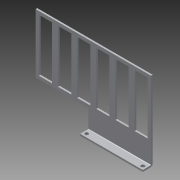
# Autodesk Inventor part: Wall
Saved by Autodesk Inventor 2013 (Build 170138000, 138)
## iProperties
Created: 2013-02-01
Part Number: Wall
Material: Aluminum 6061
Document SubType Name: Sheet Metal
Designer: actoennies
Mass: 272.717 g
Surface Area: 659.98 cm^2
Volume: 100.633 cm^3
Density: 2.71 g/cm^3
Sheet Metal Rule: Default
Author: actoennies
Autodesk Inventor part; units mm, degrees
ref_plane "YZ Plane" through (0, 0, 0) normal (1, 0, 0) x (0, 1, 0)
ref_plane "XZ Plane" through (0, 0, 0) normal (0, 1, 0) x (-1, 0, 0)
ref_plane "XY Plane" through (0, 0, 0) normal (0, 0, 1) x (1, 0, 0)
sketch "Sketch1" plane through (0, 0, 0) normal (0, 1, 0) x (-1, 0, 0)
  line L0 (0, 0) -> (0, 19.05)
  line L1 (0, 19.05) -> (120.65, 19.05)
  line L2 (120.65, 19.05) -> (120.65, 0)
  line L3 (120.65, 0) -> (0, 0)
  circle A0 centre (6.35, 12.7) radius 3.3782
  circle A1 centre (114.3, 12.7) radius 3.3782
  dimension "d0" = 19.05
  dimension "d1" = 120.65
  dimension "d2" = 6.7564
  dimension "d3" = 6.7564
  dimension "d4" = 107.95
  dimension "d5" = 6.35
  dimension "d6" = 12.7
  dimension "d7" = 12.7
  measures "d0" distance of L0.start L0.end
  measures "d1" distance of L0.end L1.end
  measures "d2" diameter of A0
  measures "d3" diameter of A1
  measures "d4" distance of A1.centre A0.centre
  measures "d5" distance from line of L0 A0.centre
  measures "d6" distance from line of L3 A0.centre
  measures "d7" distance from line of L3 A1.centre
extrude "Plate1" add sketch "Sketch1" along normal blind 3.175
sketch "Sketch2" plane through (-120.65, 0, 3.175) normal (0, 0, -1) x (-1, 0, 0)
  line L0 (-120.65, 0) -> (0, 0)
  line L1 (0, 0) -> (0, 38.1)
  line L2 (0, 38.1) -> (-120.65, 38.1)
  line L3 (-120.65, 38.1) -> (-120.65, 0)
  constraints: 6 end point, 1 horizontal, 1 perpendicular, 1 vertical
edge flange "Flange1" height 38.1 angle 90 thickness 3.175 bend radius 1.27 thickness toward (0, 0, -1) relief straight relief width 3.175 relief depth 1.5875 edges at (-60.325, 3.175, 0) wall of the first edge with corners at (0, 0, 3.175) (-120.65, 0, 3.175) (-120.65, 38.1, 3.175) (0, 38.1, 3.175)
bend "Bend1"
corner "Corner1"
sketch "Sketch3" plane through (-120.65, 38.1, 3.175) normal (0, 0, 1) x (1, 0, 0)
  line L0 (120.65, 0) -> (0, 0)
  line L1 (0, 0) -> (0, -33.655)
  line L2 (0, 0) -> (-101.6, 0)
  line L3 (-101.6, 0) -> (-101.6, 114.3)
  line L4 (-101.6, 114.3) -> (120.65, 114.3)
  line L5 (120.65, 114.3) -> (120.65, 0)
  point P0 (120.65, -38.1)
  dimension "d19" = 101.6
  dimension "d20" = 114.3
  measures "d19" distance of L0.end L2.end
  measures "d20" distance of L2.end L3.end
sheet face with bend "Face2" sketch "Sketch3" thickness 3.175 toward (0, 0, -1) bend radius 3.175 relief straight relief width 3.175 relief depth 1.5875
bend "Bend2"
sketch "Sketch4" plane through (-120.65, 4.445, 3.175) normal (0, 0, 1) x (1, 0, 0)
  line L0 (120.65, 147.955) -> (-101.6, 147.955) projected
  line L1 (-101.6, 147.955) -> (-101.6, 33.655) projected
  line L2 (-101.6, 33.655) -> (0, 33.655) projected
  line L3 (0, 33.655) -> (0, 0) projected
  line L4 (-95.25, 141.605) -> (-69.85, 141.605)
  line L5 (-69.85, 141.605) -> (-69.85, 40.005)
  line L6 (-69.85, 40.005) -> (-95.25, 40.005)
  line L7 (-95.25, 40.005) -> (-95.25, 141.605)
  line L8 (-58.42, 141.605) -> (-33.02, 141.605)
  line L9 (-33.02, 141.605) -> (-33.02, 40.005)
  line L10 (-33.02, 40.005) -> (-58.42, 40.005)
  line L11 (-58.42, 40.005) -> (-58.42, 141.605)
  line L12 (-21.59, 141.605) -> (3.81, 141.605)
  line L13 (3.81, 141.605) -> (3.81, 40.005)
  line L14 (3.81, 40.005) -> (-21.59, 40.005)
  line L15 (-21.59, 40.005) -> (-21.59, 141.605)
  line L16 (15.24, 141.605) -> (40.64, 141.605)
  line L17 (40.64, 141.605) -> (40.64, 40.005)
  line L18 (40.64, 40.005) -> (15.24, 40.005)
  line L19 (15.24, 40.005) -> (15.24, 141.605)
  line L20 (52.07, 141.605) -> (77.47, 141.605)
  line L21 (77.47, 141.605) -> (77.47, 40.005)
  line L22 (77.47, 40.005) -> (52.07, 40.005)
  line L23 (52.07, 40.005) -> (52.07, 141.605)
  line L24 (88.9, 141.605) -> (114.3, 141.605)
  line L25 (114.3, 141.605) -> (114.3, 40.005)
  line L26 (114.3, 40.005) -> (88.9, 40.005)
  line L27 (88.9, 40.005) -> (88.9, 141.605)
  point P0 (120.65, -4.445)
  dimension "d26" = 25.4
  dimension "d27" = 101.6
  dimension "d28" = 25.4
  dimension "d29" = 6.35
  dimension "d30" = 69.85
  dimension "d31" = 222.25
  dimension "d32" = 6.35
  dimension "d35" = 36.83
  constraints: 48 end point, 2 perpendicular, 1 horizontal, 1 parallel, 40 other
  measures "d26" distance of L4.start L4.end
  measures "d27" distance of L4.end L5.end
  measures "d28" distance of L5.end L6.end
  measures "d29" distance between parallel lines of L0 L4
  measures "d30" distance between parallel lines of L3 L5
  measures "d31" distance of L0.start L0.end
  measures "d32" distance from line of L4.start L1
  measures "d35" distance of L4.start L8.start
extrude "Cut1" cut sketch "Sketch4" against normal blind 3.175
equation "\"d40\" = Thickness"
equation "\"d9\" = BendReliefWidth"
equation "\"d10\" = BendReliefDepth"
equation "\"d11\" = MinimumRemnant"
equation "\"d12\" = BendRadius"
equation "\"d16\" = CornerReliefSize"
equation "\"d17\" = GapSize"
equation "\"d18\" = JacobiRadiusSize"
equation "\"d21\" = BendRadius"
equation "\"d22\" = BendReliefWidth"
equation "\"d24\" = MinimumRemnant"
equation "\"d23\" = BendReliefDepth"
equation "\"d25\" = BendRadius"
equation "\"BendRadius\" = Thickness"
equation "\"BendReliefWidth\" = Thickness"
equation "\"BendReliefDepth\" = 0.5 * Thickness"
equation "\"CornerReliefSize\" = 4 * Thickness"
equation "\"MinimumRemnant\" = 2 * Thickness"
equation "\"TransitionRadius\" = BendRadius"
equation "\"JacobiRadiusSize\" = BendRadius"
equation "\"GapSize\" = Thickness"
equation "\"d8\" = BendRadius"
equation "\"Thickness\" = 3.175"
body "Solid1"
